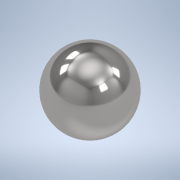
# Autodesk Inventor part: Ball
Saved by Autodesk Inventor 2022 (Build 260153000, 153)
## iProperties
Created: 2022-04-26
Part Number: Ball
Material: Generic
Document SubType Name: Modeling
Designer: Nick
Density: 1 g/cm^3
Appearance: Steel - Polished
Author: Nick
Autodesk Inventor part; units mm, degrees
ref_plane "YZ Plane" through (0, 0, 0) normal (1, 0, 0) x (0, 1, 0)
ref_plane "XZ Plane" through (0, 0, 0) normal (0, 1, 0) x (-1, 0, 0)
ref_plane "XY Plane" through (0, 0, 0) normal (0, 0, 1) x (1, 0, 0)
sketch "Sketch1" plane through (0, 0, 0) normal (0, 0, 1) x (1, 0, 0)
  circle A0 centre (0, 0) radius 6.35
  line L0 (-17.6917, 0) -> (23.0471, 0)
  point P0 (-6.35, 0)
  point P1 (6.35, 0)
  dimension "d0" = 12.7
  constraints: 2 end point, 1 centre point, 1 coincident, 1 horizontal, 1 point on line
  measures "d0" diameter of A0
revolve "Revolution1" add sketch "Sketch1" angle 360 about axis through (-17.6917, 0, 0) along (1, 0, 0) picked at (1.8268, 2.3873) contours L0 A0
body "Solid1"
